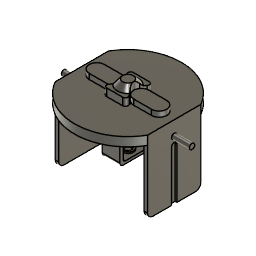
Dot Stamp (Autodesk Fusion 360 design; units mm, degrees)
Autodesk Fusion 360 part; units mm, degrees
note: some values were not read from the file. Chosen so that the rebuilt part matches the saved one: which bodies a step acts on; which face or edge a step refers to; which pieces of a blend or face edit are solid. Set by a fixed rule: which sketch regions a step uses.
sketch "Sketch2" plane through (0, 0, 0) normal (0, 0, 1) x (1, 0, 0)
  circle A0 centre (0, 0) radius 3
  line L0 (-4.5, 7.5) -> (4.5, 7.5)
  line L1 (4.5, -7.5) -> (-4.5, -7.5)
  line L2 (5.7, 5.1) -> (3.9, 2.7)
  line L3 (5.7, -5.1) -> (3.9, -2.7)
  line L4 (-5.7, -5.1) -> (-3.9, -2.7)
  line L5 (-5.7, 5.1) -> (-3.9, 2.7)
  arc A1 (-3.9, -2.7) -> (-3.9, 2.7) centre (-7.5, 0) ccw
  arc A2 (3.9, 2.7) -> (3.9, -2.7) centre (7.5, 0) ccw
  arc A3 (-4.5, 7.5) -> (-5.7, 5.1) centre (-4.5, 6) ccw
  arc A4 (5.7, 5.1) -> (4.5, 7.5) centre (4.5, 6) ccw
  arc A5 (4.5, -7.5) -> (5.7, -5.1) centre (4.5, -6) ccw
  arc A6 (-5.7, -5.1) -> (-4.5, -7.5) centre (-4.5, -6) ccw
  line L6 (-5.7, 5.1) -> (-5.7, -5.1)
  line L7 (5.7, 5.1) -> (5.7, -5.1)
  point P0 (-7.5, 7.5)
  point P1 (7.5, 7.5)
  point P2 (7.5, -7.5)
  point P3 (-7.5, -7.5)
  dimension "d22" = 6
  dimension "d23" = 9
  dimension "d24" = 9
  dimension "d25" = 15
  dimension "d26" = 15
  dimension "d27" = 15
  dimension "d28" = 7.5
  dimension "d29" = 1.5
  dimension "d30" = 1.5
  constraint coincident A0.centre origin
  constraint horizontal L0
  constraint horizontal L1
  constraint tangent L2 A2
  constraint tangent L3 A2
  constraint tangent L4 A1
  constraint parallel L2 L4
  constraint tangent L5 A1
  constraint tangent A0 A1
  constraint tangent A0 A2
  constraint vertical P1 P2
  constraint collinear A0.centre A2.centre A1.centre
  constraint horizontal A0.centre A2.centre
  constraint coincident P0 L0
  constraint coincident P0 L5
  constraint tangent L0 A3
  constraint tangent L5 A3
  constraint coincident P1 L0
  constraint coincident P1 L2
  constraint tangent L0 A4
  constraint tangent L2 A4
  constraint coincident P2 L1
  constraint coincident P2 L3
  constraint tangent L1 A5
  constraint tangent L3 A5
  constraint equal A4 A5
  constraint coincident P3 L1
  constraint coincident P3 L4
  constraint tangent L1 A6
  constraint tangent L4 A6
  constraint equal A4 A6
  measures "d22" diameter of A0
  measures "d23" diameter of A2
  measures "d24" diameter of A1
  measures "d25" distance of P0 P1
  measures "d26" distance of P2 P3
  measures "d27" distance of L0 L1
  measures "d28" distance of A0.centre L0
  measures "d29" radius of A3
  measures "d30" radius of A4
extrude "Extrude3" add sketch "Sketch2" along normal blind 5 contours A0 | A0 L1 L3 L4 A1 A2 A5 A6 | A0 L0 L2 L5 A1 A2 A3 A4 makes body 1
extrude "Extrude4" add sketch "Sketch2" along normal blind 3 from surface at 5 contours A0 bodies 1
extrude "Extrude5" add sketch "Sketch2" against normal blind 1 bodies 1
sketch "Sketch3" plane through (0, 0, 0) normal (0, 0, 1) x (1, 0, 0)
  line L0 (-5.7, 5.1) -> (-5.7, -5.1) construction
  arc A0 (-4.5, 7.5) -> (-5.7, 5.1) centre (-4.5, 6) ccw construction
  line L1 (-4.5, 7.5) -> (4.5, 7.5) construction
  line L2 (-5.7, 5.1) -> (-3.9, 2.7) construction
  arc A1 (-3.9, -2.7) -> (-3.9, 2.7) centre (-7.5, 0) ccw construction
  line L3 (-5.7, -5.1) -> (-3.9, -2.7) construction
  arc A2 (-5.7, -5.1) -> (-4.5, -7.5) centre (-4.5, -6) ccw construction
  line L4 (4.5, -7.5) -> (-4.5, -7.5) construction
  arc A3 (4.5, -7.5) -> (5.7, -5.1) centre (4.5, -6) ccw construction
  line L5 (5.7, 5.1) -> (5.7, -5.1) construction
  line L6 (5.7, -5.1) -> (3.9, -2.7) construction
  arc A4 (3.9, 2.7) -> (3.9, -2.7) centre (7.5, 0) ccw construction
  line L7 (5.7, 5.1) -> (3.9, 2.7) construction
  arc A5 (5.7, 5.1) -> (4.5, 7.5) centre (4.5, 6) ccw construction
  line L8 (0, 7.5) -> (0, -7.525) construction
  line L9 (-25.9808, 15) -> (-25.9808, -15)
  line L10 (25.9808, 15) -> (25.9808, -15)
  arc A6 (25.9808, 15) -> (-25.9808, 15) centre (0, 0) ccw
  arc A7 (-25.9808, -15) -> (25.9808, -15) centre (0, 0) ccw
  line L11 (-5.86, -4.98) -> (-4.06, -2.58)
  arc A8 (-4.06, -2.58) -> (-4.06, 2.58) centre (-7.5, 0) ccw
  line L12 (-5.86, 4.98) -> (-4.06, 2.58)
  arc A9 (-4.5, 7.7) -> (-5.86, 4.98) centre (-4.5, 6) ccw
  line L13 (-4.5, 7.7) -> (4.5, 7.7)
  arc A10 (5.86, 4.98) -> (4.5, 7.7) centre (4.5, 6) ccw
  line L14 (5.86, 4.98) -> (4.06, 2.58)
  arc A11 (4.06, 2.58) -> (4.06, -2.58) centre (7.5, 0) ccw
  line L15 (5.86, -4.98) -> (4.06, -2.58)
  arc A12 (4.5, -7.7) -> (5.86, -4.98) centre (4.5, -6) ccw
  line L16 (4.5, -7.7) -> (-4.5, -7.7)
  arc A13 (-5.86, -4.98) -> (-4.5, -7.7) centre (-4.5, -6) ccw
  line L17 (-17.5, 4.3) -> (-7.5, 4.3)
  line L18 (-17.5, -4.3) -> (-7.5, -4.3)
  line L19 (7.5, -4.3) -> (17.5, -4.3)
  line L20 (7.5, 4.3) -> (17.5, 4.3)
  arc A14 (-17.5, 4.3) -> (-17.5, -4.3) centre (-17.5, 0) ccw
  arc A15 (-7.5, -4.3) -> (-7.5, 4.3) centre (-7.5, 0) ccw
  arc A16 (7.5, 4.3) -> (7.5, -4.3) centre (7.5, 0) ccw
  arc A17 (17.5, -4.3) -> (17.5, 4.3) centre (17.5, 0) ccw
  line L21 (-5.9, -3.9912) -> (-5.9, -5.0356)
  line L22 (5.8, -3.9497) -> (5.8, -4.9046)
  line L23 (5.8, 4.9046) -> (5.8, 3.9497)
  line L24 (-5.8, 4.9046) -> (-5.8, 3.9497)
  dimension "d44" = 30
  dimension "d46" = 30
  dimension "d47" = 30
  dimension "d122" = -0.2
  dimension "d123" = 30
  dimension "d124" = 10
  dimension "d125" = 10
  dimension "d126" = 0.1
  dimension "d127" = 0.1
  dimension "d128" = 0.2
  dimension "d130" = 0.1
  constraint coincident A6.centre A7.centre
  constraint vertical L9
  constraint concentric A1 A15
  constraint concentric A4 A16
  constraint equal A8 A15
  constraint equal A11 A16
  constraint coincident L10 A6.start
  constraint coincident L10 A7.end
  constraint vertical L10
  constraint coincident L10.start A6.start
  constraint coincident L10.end A7.end
  constraint equal A14 A15
  constraint equal A15 A17
  constraint horizontal A4.centre A17.centre
  constraint horizontal A1.centre A14.centre
  constraint tangent L18 A15
  constraint tangent L19 A17
  constraint tangent L20 A17
  constraint tangent L19 A16
  constraint tangent L20 A16
  constraint tangent L17 A15
  constraint tangent L17 A14
  constraint tangent L18 A14
  constraint coincident A15 L21.start
  constraint coincident A13 L21.end
  constraint vertical L21
  constraint coincident A16 L22.start
  constraint coincident A12 L22.end
  constraint parallel L21 L22
  constraint coincident A10 L23.start
  constraint coincident A16 L23.end
  constraint parallel L22 L23
  constraint coincident A9 L24.start
  constraint coincident A15 L24.end
  constraint vertical L24
  measures "d44" radius of A7
  measures "d46" distance of L9.start L9.end
  measures "d47" distance of L10.start L10.end
  measures "d123" radius of A6
  measures "d124" distance of A1.centre A14.centre
  measures "d125" distance of A4.centre A17.centre
  measures "d126" distance of L5 L23
  measures "d127" distance of L5 L22
  measures "d128" distance of L0 L21
  measures "d130" distance of L0 L24
extrude "Extrude6" add sketch "Sketch3" along normal blind 1 separate body makes body 2
extrude "Extrude7" add sketch "Sketch3" against normal blind 4 bodies 2
extrude "Extrude23" add sketch "Sketch3" along normal blind 3 from surface at 1 contours A8 L17 L18 A14 A15 | A11 L19 L20 A16 A17 bodies 2
sketch "Sketch4" plane through (0, 0, -1) normal (0, 0, -1) x (1, 0, 0)
  arc A0 (-5.7, -5.1) -> (-4.5, -7.5) centre (-4.5, -6) ccw
  line L0 (-4.5, -7.5) -> (4.5, -7.5)
  arc A1 (4.5, -7.5) -> (5.7, -5.1) centre (4.5, -6) ccw
  line L1 (5.7, -5.1) -> (5.7, 5.1)
  arc A2 (5.7, 5.1) -> (4.5, 7.5) centre (4.5, 6) ccw
  line L2 (4.5, 7.5) -> (-4.5, 7.5)
  arc A3 (-4.5, 7.5) -> (-5.7, 5.1) centre (-4.5, 6) ccw
  line L3 (-5.7, 5.1) -> (-5.7, -5.1)
  circle A4 centre (0, 0) radius 2.1
  circle A5 centre (0, 0) radius 3.1
  dimension "d63" = 4.2
  dimension "d64" = 1
  constraint coincident A4.centre A5.centre
  measures "d63" diameter of A4
extrude "Extrude11" cut sketch "Sketch4" against normal blind 0.5 contours A4 bodies 1
extrude "Extrude12" add sketch "Sketch4" along normal blind 1 contours A5 bodies 1
extrude "Extrude13" add 1 faces at (2.7473, 0.2583, -2) along direction (0, 0, 1) blind 1.5 from surface at -25 separate body on bodies 1 makes body 3
ref_plane "WorkPlane1" through (0, 0, -26.25) normal (0, 0, -1) x (1, 0, 0)
sketch "Sketch5" plane through (0, 0, -26.25) normal (0, 0, -1) x (-1, 0, 0)
  circle A0 centre (0, 0) radius 2.1
  circle A1 centre (0, 0) radius 3.1
  circle A2 centre (0, 0) radius 3.1
  arc A3 (5.7, 5.1) -> (4.5, 7.5) centre (4.5, 6) ccw
  line L0 (4.5, 7.5) -> (-4.5, 7.5)
  arc A4 (-4.5, 7.5) -> (-5.7, 5.1) centre (-4.5, 6) ccw
  line L1 (-5.7, 5.1) -> (-5.7, -5.1) construction
  arc A5 (-5.7, -5.1) -> (-4.5, -7.5) centre (-4.5, -6) ccw
  line L2 (-4.5, -7.5) -> (4.5, -7.5)
  arc A6 (4.5, -7.5) -> (5.7, -5.1) centre (4.5, -6) ccw
  line L3 (5.7, -5.1) -> (5.7, 5.1) construction
  arc A7 (25.9808, 15) -> (-25.9808, 15) centre (0, 0) ccw
  line L4 (25.9808, -15) -> (25.9808, 15)
  line L5 (-25.9808, 15) -> (-25.9808, -15)
  arc A8 (-25.9808, -15) -> (25.9808, -15) centre (0, 0) ccw
  circle A9 centre (0, 14) radius 1.5
  line L6 (-5, 18) -> (5, 18)
  line L7 (5, 18) -> (5, 7.6)
  line L8 (-5, 7.6) -> (-5, 18)
  line L9 (-5, 9.6) -> (5, 9.6)
  line L10 (-5, 7.6) -> (5, 7.6)
  line L11 (5, 7.6) -> (5, -7.6)
  line L12 (5, -7.6) -> (-5, -7.6)
  line L13 (-5, -7.6) -> (-5, 7.6)
  line L14 (0, 0) -> (8, 0) construction
  circle A10 centre (0, -14) radius 1.5
  line L15 (-5, -7.6) -> (-5, -18)
  line L16 (-5, -9.6) -> (5, -9.6)
  line L17 (-5, -18) -> (5, -18)
  line L18 (5, -18) -> (5, -7.6)
  line L19 (-7.5, -4.3) -> (-17.5, -4.3)
  arc A11 (-17.5, 4.3) -> (-17.5, -4.3) centre (-17.5, 0) ccw
  line L20 (-17.5, 4.3) -> (-7.5, 4.3)
  arc A12 (-7.5, -4.3) -> (-5.8, -3.9497) centre (-7.5, 0) ccw
  line L21 (7.5, 4.3) -> (17.5, 4.3)
  arc A13 (17.5, -4.3) -> (17.5, 4.3) centre (17.5, 0) ccw
  line L22 (17.5, -4.3) -> (7.5, -4.3)
  arc A14 (7.5, 4.3) -> (5.8, 3.9497) centre (7.5, 0) ccw
  line L23 (5, -7.6) -> (-5, 7.6) construction
  arc A15 (5.86, 4.98) -> (4.5, 7.7) centre (4.5, 6) ccw
  line L24 (5.86, 4.98) -> (5.8, 4.9)
  line L25 (5.8, 4.9) -> (5.8, 3.9497)
  arc A16 (5.9, -3.9912) -> (7.5, -4.3) centre (7.5, 0) ccw
  line L26 (5.9, -3.9912) -> (5.9, -5.0356)
  arc A17 (4.5, -7.7) -> (5.9, -5.0356) centre (4.5, -6) ccw
  line L27 (4.5, -7.7) -> (-4.5, -7.7)
  arc A18 (-5.86, -4.98) -> (-4.5, -7.7) centre (-4.5, -6) ccw
  line L28 (-5.86, -4.98) -> (-5.8, -4.9)
  line L29 (-5.8, -4.9) -> (-5.8, -3.9497)
  arc A19 (-5.8, 3.9497) -> (-7.5, 4.3) centre (-7.5, 0) ccw
  line L30 (-5.8, 3.9497) -> (-5.8, 4.9)
  line L31 (-5.8, 4.9) -> (-5.86, 4.98)
  arc A20 (-4.5, 7.7) -> (-5.86, 4.98) centre (-4.5, 6) ccw
  line L32 (-4.5, 7.7) -> (4.5, 7.7)
  dimension "d72" = 3
  dimension "d73" = 14
  dimension "d74" = 2
  dimension "d75" = 4
  dimension "d76" = 8
  dimension "d131" = 10
  dimension "d132" = 7.6
  constraint horizontal L6
  constraint vertical L7
  constraint vertical L8
  constraint coincident L8 L9.start
  constraint coincident L7 L9.end
  constraint perpendicular L7 L9
  constraint horizontal L10
  constraint vertical L11
  constraint horizontal L12
  constraint vertical L13
  constraint collinear L8 L13
  constraint collinear L7 L11
  constraint vertical A0.centre A9.centre
  constraint coincident L8.start L10.start
  constraint coincident L7.end L10.end
  constraint coincident A0.centre A1.centre
  constraint perpendicular L1 L14
  constraint symmetric A9 L14 A10
  constraint symmetric L6.start L14 L15.end
  constraint symmetric L6.end L14 L17.end
  constraint symmetric L7.end L14 L11.end
  constraint symmetric L8.start L14 L12.end
  constraint symmetric L9.start L14 L16.start
  constraint symmetric L9.end L14 L16.end
  constraint midpoint A0.centre L23
  constraint coincident L11.end L12.start
  measures "d72" diameter of A9
  measures "d73" distance of A0.centre A9.centre
  measures "d74" distance of L9 L10
  measures "d75" distance of A9.centre L6
  measures "d76" distance of A0.centre L14.end
  measures "d131" distance of L6.start L6.end
  measures "d132" distance of A0.centre L10
extrude "Extrude14" cut sketch "Sketch5" against normal blind 2 from surface at -22.25 contours A9 | A10 bodies 2
extrude "Extrude15" add sketch "Sketch5" along normal blind 0.5 contours A3 L0 A4 A5 L2 A6 L11 L13 | A3 L0 A4 L10 L11 L13 | A5 L2 A6 L11 L12 L13 bodies 3
extrude "Extrude16" add sketch "Sketch5" along normal blind 1 from surface at 0.5 contours A0 | A1 A2 | A3 L0 A4 A5 L2 A6 L11 L13 | A3 L0 A4 L10 L11 L13 | A5 L2 A6 L11 L12 L13 bodies 3
extrude "Extrude17" add sketch "Sketch5" along normal up to surface (23.75 mm away) from surface at -22.25 separate body contours L7 L8 L10 A15 A20 L32 | L7 L8 L9 A15 A20 L32 | L12 L15 L18 A17 L27 A18 | L15 L16 L18 A17 L27 A18 makes body 4 at (-1.6667, -9.6, -19.8333) makes body 5 at (-1.6667, 7.6, -19.8333)
extrude "Extrude18" add sketch "Sketch5" against normal blind 2 draft -10 from surface at -22.25 separate body contours A9 | A10 makes body 6 at (-0.7108, 12.7688, -3.5556) makes body 7 at (-0.7108, -15.2312, -3.5556)
extrude "Extrude19" add sketch "Sketch5" along normal blind 1 from surface at -22.25 separate body contours L6 L7 L8 L9 | L15 L16 L17 L18 | A9 | A10 makes body 8 at (1.6667, -15.2, -4) makes body 9 at (-1.6667, 12.4, -4)
combine "Combine1" operation add target body 4 tool bodies 8 3
combine "Combine2" operation add target body 4 tool bodies 7 9 5 6
fillet "Fillet1" radius 2 2 edges at (0, 9.6, -27.75) (0, -9.6, -27.75) on bodies 4
fillet "Fillet2" radius 1 2 edges at (0, 7.6, -26.25) (0, -7.6, -26.25) on bodies 4
chamfer "Chamfer2" distance 4 distance2 8.4 1 edges at (0, -9.6, -5) measured on face at (1.6667, -9.6, -11.9167) on bodies 4
chamfer "Chamfer3" distance 8.4 distance2 4 1 edges at (0, 9.6, -5) measured on face at (-1.6667, 12.4, -5) on bodies 4
ref_plane "WorkPlane2" through (-25.9808, 0, -1.5) normal (-1, 0, 0) x (0, -1, 0)
sketch "Sketch6" plane through (-25.9808, 0, 0) normal (-1, 0, 0) x (0, -1, 0)
  line L0 (15, -4) -> (15, 1) construction
  line L1 (15, 1) -> (-15, 1) construction
  line L2 (-15, -4) -> (15, -4)
  line L3 (-15, -4) -> (-15, -37)
  line L4 (15, -4) -> (15, -37)
  line L5 (12, -40) -> (-12, -40)
  line L6 (-1.5, -40) -> (1.5, -40)
  line L7 (1.5, -40) -> (1.5, -11.5)
  line L8 (-1.5, -11.5) -> (-1.5, -40)
  arc A0 (1.5, -11.5) -> (-1.5, -11.5) centre (0, -11.5) ccw
  circle A1 centre (0, -7) radius 1.5
  arc A2 (-15, -37) -> (-12, -40) centre (-12, -37) ccw
  arc A3 (12, -40) -> (15, -37) centre (12, -37) ccw
  line L9 (-15, 1) -> (-15, -4)
  point P0 (-15, -40)
  dimension "d105" = 36
  dimension "d107" = 3
  dimension "d108" = 28.5
  dimension "d109" = 3
  dimension "d110" = 4.5
  dimension "d111" = 3
  dimension "d112" = 3
  constraint coincident L2.start L3.start
  constraint perpendicular L2 L3
  constraint coincident L0.start L2.end
  constraint perpendicular L2 L4
  constraint horizontal L5
  constraint horizontal L6
  constraint vertical L7
  constraint vertical L8
  constraint coincident L5 L6.start
  constraint tangent L7 A0
  constraint tangent L8 A0
  constraint coincident L5 L6
  constraint coincident P0 L3
  constraint coincident P0 L5
  constraint tangent L3 A2
  constraint tangent L5 A2
  constraint tangent L4 A3
  constraint tangent L5 A3
  constraint midpoint L5 L6
  constraint vertical A0.centre A1.centre
  measures "d105" distance of L2.start P0
  measures "d107" distance of L6.start L6.end
  measures "d108" distance of L6.end L7.end
  measures "d109" diameter of A1
  measures "d110" distance of A0.centre A1.centre
  measures "d111" radius of A2
  measures "d112" radius of A3
extrude "Extrude20" add sketch "Sketch6" against normal blind 1 contours L2 L3 L4 L5 L7 L8 A0 A2 A3 | A1 bodies 2
extrude "Extrude21" add sketch "Sketch6" against normal blind 1 from surface at -1 contours L2 L3 L4 L5 L7 L8 A0 A2 A3 | L5 L6 L7 L8 A0 | A1 bodies 2
extrude "Extrude22" add sketch "Sketch6" along normal blind 10 contours A1 bodies 2
mirror "Mirror1" about plane through (0, 0, 0) normal (1, 0, 0) of "Extrude20", "Extrude21", "Extrude22"
chamfer "Chamfer1" distance 3 angle 45 2 edges at (0, -3, 5) (0, 3, 5) on bodies 1
chamfer "Chamfer4" distance 1 angle 45 1 edges at (-2.8902, -1.121, -1) on bodies 1
sketch "Sketch1" plane through (0, 0, 0) normal (0, 0, 1) x (1, 0, 0)
  line L0 (0.8346, 2.5) -> (2.5, 2.5)
  line L1 (2.5, 2.5) -> (2.5, -2.5)
  line L2 (-2.5, -2.5) -> (-2.5, 2.5)
  line L3 (-2.5, 2.5) -> (2.5, -2.5) construction
  line L4 (2.5, 0) -> (0, 0) construction
  line L5 (2.5, 0.75) -> (1.75, 0.75)
  line L6 (2.5, -0.75) -> (1.75, -0.75)
  arc A0 (1.75, 0.75) -> (1.75, -0.75) centre (1.75, 0) ccw
  line L7 (-0.6709, 2.8149) -> (-0.9956, 3.2777)
  line L8 (-0.75, 3.75) -> (0.75, 3.75)
  line L9 (0.9956, 3.2777) -> (0.6709, 2.8149)
  line L10 (0, 3.75) -> (0, 2.5) construction
  arc A1 (-0.75, 3.75) -> (-0.9956, 3.2777) centre (-0.75, 3.45) ccw
  arc A2 (0.9956, 3.2777) -> (0.75, 3.75) centre (0.75, 3.45) ccw
  arc A3 (0.6709, 2.8149) -> (0.8346, 2.5) centre (0.8346, 2.7) ccw
  line L11 (-0.8346, 2.5) -> (-2.5, 2.5)
  arc A4 (-0.8346, 2.5) -> (-0.6709, 2.8149) centre (-0.8346, 2.7) ccw
  line L12 (0.8346, -2.5) -> (2.5, -2.5)
  arc A5 (0.8346, -2.5) -> (0.6709, -2.8149) centre (0.8346, -2.7) ccw
  line L13 (0.9956, -3.2777) -> (0.6709, -2.8149)
  arc A6 (0.75, -3.75) -> (0.9956, -3.2777) centre (0.75, -3.45) ccw
  line L14 (-0.75, -3.75) -> (0.75, -3.75)
  arc A7 (-0.9956, -3.2777) -> (-0.75, -3.75) centre (-0.75, -3.45) ccw
  line L15 (-0.6709, -2.8149) -> (-0.9956, -3.2777)
  arc A8 (-0.6709, -2.8149) -> (-0.8346, -2.5) centre (-0.8346, -2.7) ccw
  line L16 (-0.8346, -2.5) -> (-2.5, -2.5)
  point P0 (-0.45, 2.5)
  point P1 (-1.3269, 3.75)
  point P2 (1.3269, 3.75)
  point P3 (0.45, 2.5)
  dimension "d1" = 5
  dimension "d2" = 5
  dimension "d4" = 0.75
  dimension "d5" = 0.75
  dimension "d9" = 1.25
  dimension "d10" = 0.3
  dimension "d11" = 0.3
  dimension "d12" = 0.2
  dimension "d13" = 0.2
  dimension "d14" = 1.5
  dimension "d15" = 2.5
  dimension "d16" = 0.9
  constraint horizontal L0
  constraint vertical L1
  constraint vertical L2
  constraint midpoint L4.end L3
  constraint midpoint L1 L4.start
  constraint coincident L4.end origin
  constraint coincident A0.centre L4
  constraint coincident L1 L5.start
  constraint tangent L5 A0
  constraint coincident L1 L6.start
  constraint tangent L6 A0
  constraint perpendicular L1 L6
  constraint perpendicular L1 L5
  constraint coincident L0 P0
  constraint coincident L0 P3
  constraint perpendicular L0 L10
  constraint horizontal L8
  constraint coincident L8 L10.start
  constraint coincident P1 L7
  constraint coincident P1 L8
  constraint tangent L7 A1
  constraint tangent L8 A1
  constraint coincident P2 L8
  constraint coincident P2 L9
  constraint tangent L8 A2
  constraint tangent L9 A2
  constraint coincident L0 L10.end
  constraint coincident L2.end L0
  constraint coincident P3 L9
  constraint tangent L0 A3
  constraint tangent L9 A3
  constraint coincident P0 L7
  constraint coincident P0 L11
  constraint tangent L7 A4
  constraint tangent L11 A4
  constraint equal L0 L11
  constraint midpoint L8 L10.start
  constraint perpendicular L2 L11
  constraint symmetric L2.end L4 L2.start
  constraint symmetric L0.end L4 L1.end
  constraint symmetric L4 L7.end A7.start
  constraint symmetric L4 L8.start L14.start
  constraint symmetric L4 A1 A7
  constraint symmetric L4 L8.end A6.start
  constraint symmetric L4 L9.start L13.start
  constraint symmetric L4 A2 A6
  constraint symmetric L4 L0.start L12.start
  constraint symmetric L4 L9.end A5.end
  constraint symmetric L4 A3 A5
  constraint symmetric L4 L7.start L15.start
  constraint symmetric L4 L11.start A8.end
  constraint symmetric L4 A4 A8
  measures "d1" distance of L2.end L0.end
  measures "d2" distance of L2.end L2.start
  measures "d4" distance of A0.centre L4.start
  measures "d5" radius of A0
  measures "d9" distance of L10.start L10.end
  measures "d10" radius of A1
  measures "d11" radius of A2
  measures "d12" radius of A3
  measures "d13" radius of A4
  measures "d14" distance of L8.start L8.end
  measures "d15" distance of L1 L10
  measures "d16" distance of P0 P3
extrude "Extrude1" [suppressed]
extrude "Extrude2" [suppressed]
equation "d15 = d1 / 2"
equation "d23 = d24"
equation "d26 = d25"
equation "d27 = d25"
equation "d28 = d27 / 2"
equation "d29 = d30"
equation "d45 = d44"
equation "d46 = d45"
equation "d47 = d46"
equation "d107 = d109"
equation "d108 = 9.5 mm * 3"
equation "d110 = 1.5 * 3 mm"
equation "d123 = d44"
